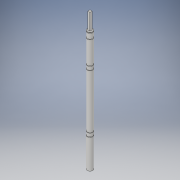
# Autodesk Inventor part: Förderbandwelle_vorne
Saved by Autodesk Inventor 2018 (Build 220112000, 112)
## iProperties
Created: 2017-12-01
Part Number: Förderbandwelle_vorne
Material: Generisch
Document SubType Name: Modeling
Designer: Dominik
Density: 1 g/cm^3
Appearance: Vorgabe
Author: Dominik
Autodesk Inventor part; units mm, degrees
sketch "Skizze1" plane through (0, 0, 0) normal (0, 0, 1) x (1, 0, 0)
  circle A0 centre (0, 0) radius 5
  dimension "d0" = 10
  constraints: 1 centre point, 1 coincident
  measures "d0" diameter of A0
extrude "Extrusion1" add sketch "Skizze1" along normal blind 140
sketch "Skizze4" plane through (0, 0, 0) normal (0, 0, -1) x (-1, 0, 0)
  circle A0 centre (0, 0) radius 5
  dimension "d15" = 10
  constraints: 1 centre point, 1 coincident
  measures "d15" diameter of A0
extrude "Extrusion4" add sketch "Skizze4" along normal blind 50
sketch "Skizze5" plane through (0, 0, 140) normal (0, 0, 1) x (1, 0, 0)
  circle A0 centre (0, 0) radius 5
  constraints: 1 centre point, 1 coincident
sketch "Skizze6" plane through (0, 0, 140) normal (0, 0, 1) x (1, 0, 0)
  point P0 (0, 0)
extrude "Extrusion5" add sketch "Skizze5" along normal blind 30
sketch "Skizze7" plane through (0, 0, 170) normal (0, 0, 1) x (1, 0, 0)
  line L0 (0, 0) -> (0, 2)
  line L1 (0, 2) -> (2, 2)
  line L2 (2, 2) -> (2, -2)
  line L3 (2, -2) -> (-2, -2)
  line L4 (-2, -2) -> (-2, 2)
  line L5 (-2, 2) -> (0, 2)
  dimension "d20" = 2
  dimension "d21" = 2
  dimension "d22" = 4
  dimension "d23" = 4
  constraints: 12 end point, 4 perpendicular, 1 collinear, 1 point on line, 1 vertical
  measures "d20" distance of L0.start L0.end
  measures "d21" distance of L0.end L1.end
  measures "d22" distance of L1.end L2.end
  measures "d23" distance of L2.end L3.end
extrude "Extrusion6" add sketch "Skizze7" along normal blind 30
ref_plane "Arbeitsebene1" through (0, 5, 0) normal (0, 1, 0) x (-1, 0, 0)
sketch "Skizze8" plane through (0, 5, 0) normal (0, 1, 0) x (-1, 0, 0)
  line L0 (-5, -50) -> (5, -50) projected
  line L1 (0, -50) -> (0, 170)
  line L2 (5, 170) -> (-5, 170) projected
  line L3 (0, 170) -> (0, 60)
  line L4 (0, 60) -> (0, 112.85)
  line L5 (0, 60) -> (0, 7.15)
  line L6 (0, 8.65) -> (0, 5.65) construction
  line L7 (-1.5, 8.65) -> (-1.5, 5.65)
  line L8 (1.5, 5.65) -> (1.5, 8.65)
  arc A0 (1.5, 8.65) -> (-1.5, 8.65) centre (0, 8.65) ccw
  arc A1 (-1.5, 5.65) -> (1.5, 5.65) centre (0, 5.65) ccw
  line L9 (0, 111.35) -> (0, 114.35) construction
  line L10 (-1.5, 111.35) -> (-1.5, 114.35)
  line L11 (1.5, 114.35) -> (1.5, 111.35)
  arc A2 (-1.5, 111.35) -> (1.5, 111.35) centre (0, 111.35) ccw
  arc A3 (1.5, 114.35) -> (-1.5, 114.35) centre (0, 114.35) ccw
  point P0 (0, 0)
  dimension "d27" = 52.85
  dimension "d28" = 52.85
  dimension "d30" = 3
  dimension "d31" = 6
  dimension "d35" = 1.5
  dimension "d46" = 6
  constraints: 24 end point, 8 point on circle, 8 tangent, 5 midpoint, 4 centre point, 4 point on line, 2 parallel
  measures "d27" distance of L3.end L4.end
  measures "d28" distance of L3.end L5.end
  measures "d30" diameter of A1
  measures "d35" radius of A3
extrude "Extrusion7" cut sketch "Skizze8" against normal blind 1.5 contours A1 L7 A0 L1 | L1 A0 L8 A1
extrude "Extrusion8" cut sketch "Skizze8" against normal blind 1.5 contours A2 L10 A3 L1 | L1 A3 L11 A2
ref_plane "Arbeitsebene2" through (0, 5, 115.85) normal (0, 0, 1) x (1, 0, 0)
sketch "Skizze9" plane through (0, 5, 115.85) normal (0, 0, 1) x (1, 0, 0)
  circle A0 centre (0, -5) radius 3.8
  circle A1 centre (0, -5) radius 5
  point P0 (0, -5)
  dimension "d38" = 7.6
  dimension "d41" = 10
  constraints: 2 centre point, 2 coincident
  measures "d38" diameter of A0
  measures "d41" diameter of A1
extrude "Extrusion9" cut sketch "Skizze9" along normal blind 0.9
ref_plane "Arbeitsebene3" through (0, 5, 4.15) normal (0, 0, -1) x (-1, 0, 0)
sketch "Skizze10" plane through (0, 5, 4.15) normal (0, 0, -1) x (-1, 0, 0)
  circle A0 centre (0, -5) radius 5
  circle A1 centre (0, -5) radius 3.8
  point P0 (0, -5)
  dimension "d42" = 7.6
  constraints: 2 centre point, 2 coincident
  measures "d42" diameter of A1
extrude "Extrusion10" cut sketch "Skizze10" along normal blind 0.9
ref_plane "Arbeitsebene4" through (0, 5, 109.85) normal (0, 0, 1) x (1, 0, 0)
sketch "Skizze11" plane through (0, 5, 109.85) normal (0, 0, 1) x (1, 0, 0)
  circle A0 centre (0, -5) radius 5.4286
  circle A1 centre (0, -5) radius 3.8
  point P0 (0, -5)
  dimension "d48" = 7.6
  constraints: 2 centre point, 2 coincident
  measures "d48" diameter of A1
extrude "Extrusion11" cut sketch "Skizze11" against normal blind 0.9
ref_plane "Arbeitsebene5" through (0, 5, 10.15) normal (0, 0, -1) x (-1, 0, 0)
sketch "Skizze12" plane through (0, 5, 10.15) normal (0, 0, -1) x (-1, 0, 0)
  circle A0 centre (0, -5) radius 5.0141
  circle A1 centre (0, -5) radius 3.8
  point P0 (0, -5)
  dimension "d52" = 7.6
  constraints: 2 centre point, 2 coincident
  measures "d52" diameter of A1
extrude "Extrusion12" cut sketch "Skizze12" against normal blind 0.9
ref_plane "Arbeitsebene6" through (0, 0, 168.9) normal (0, 0, 1) x (1, 0, 0)
sketch "Skizze13" plane through (0, 0, 168.9) normal (0, 0, 1) x (1, 0, 0)
  circle A0 centre (0, 0) radius 3.8
  circle A1 centre (0, 0) radius 5
  dimension "d56" = 7.6
  dimension "d64" = 10
  constraints: 2 centre point, 2 coincident
  measures "d56" diameter of A0
  measures "d64" diameter of A1
extrude "Extrusion13" cut sketch "Skizze13" against normal blind 0.9
ref_plane "Arbeitsebene7" through (0, 0, 159) normal (0, 0, 1) x (1, 0, 0)
sketch "Skizze14" plane through (0, 0, 159) normal (0, 0, 1) x (1, 0, 0)
  circle A0 centre (0, 0) radius 5
  circle A1 centre (0, 0) radius 3.8
  dimension "d60" = 10
  dimension "d61" = 7.6
  constraints: 2 centre point, 2 coincident
  measures "d60" diameter of A0
  measures "d61" diameter of A1
extrude "Extrusion14" cut sketch "Skizze14" against normal blind 0.9
